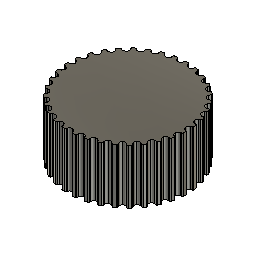
gear_35z (Autodesk Fusion 360 design; units mm, degrees)
Autodesk Fusion 360 part; units mm, degrees
sketch "Sketch1" plane through (0, 0, 0) normal (0, 0, 1) x (1, 0, 0) in component "gt2 pulley"
  circle A0 centre (0, 0) radius 11.1408 construction
  circle A1 centre (0, 0) radius 10.1368 construction
  line L0 (0, 0) -> (0, 11.1408) construction
  line L1 (0, 0) -> (0.9987, 11.096) construction
  line L2 (0, 0) -> (1.4093, 11.0514) construction
  circle A2 centre (0, 0) radius 10.8868 construction
  arc A3 (0.3788, 10.7429) -> (0.4362, 10.461) centre (1.3772, 10.7994) ccw
  circle A4 centre (0, 0) radius 10.7368 construction
  arc A5 (0.2321, 10.8844) -> (0, 10.8868) centre (0, 0) ccw
  arc A6 (0.3788, 10.7429) -> (0.2321, 10.8844) centre (0.229, 10.7344) ccw
  arc A7 (0.4362, 10.461) -> (0.9087, 10.096) centre (0.9584, 10.6488) ccw
  arc A8 (0, 10.8868) -> (-0.2321, 10.8844) centre (0, 0) ccw
  arc A9 (-0.2321, 10.8844) -> (-0.3788, 10.7429) centre (-0.229, 10.7344) ccw
  arc A10 (-0.4362, 10.461) -> (-0.3788, 10.7429) centre (-1.3772, 10.7994) ccw
  arc A11 (-0.9096, 10.096) -> (-0.4362, 10.461) centre (-0.9584, 10.6488) ccw
  arc A12 (0.9087, 10.096) -> (-0.9087, 10.096) centre (0, 0) ccw
  point P0 (1.3772, 10.7994)
  point P1 (0, 10.8868)
  dimension "d18" = 22.2817
  dimension "d19" = 5.143
  dimension "d22" = 1.004
  dimension "d24" = 0.75
  dimension "d26" = 1
  dimension "d27" = 0.15
  dimension "d28" = 0.15
  dimension "d47" = 0.555
  dimension "d52" = 3.812
  constraint coincident A0.centre A1.centre
  constraint coincident A0 L0.end
  constraint vertical L0
  constraint coincident A0 L1.end
  constraint coincident A0 L2.end
  constraint concentric A1 A2
  constraint coincident A1 A7.end
  constraint coincident L1 A7.end
  constraint coincident A2 P0
  constraint coincident L2 P0
  constraint coincident P0 A3.centre
  constraint coincident A2 P1
  constraint coincident L0 P1
  constraint concentric A2 A4
  constraint coincident P1 A5.end
  constraint coincident A4 A6.centre
  constraint coincident A3.start A6.start
  constraint tangent A3 A6
  constraint tangent A3 A7
  constraint symmetric L0 A7.end A12.end
  constraint symmetric L0 A3.start A9.end
  constraint symmetric L0 A3.end A10.start
  constraint symmetric L0 A3 A10
  constraint symmetric L0 A5.start A8.end
  constraint symmetric L0 P1 A5.end
  constraint symmetric L0 A5 A8
  constraint symmetric L0 A6 A9
  constraint symmetric L0 A7 A11
  constraint coincident A1 A11.start
  constraint tangent A1 A7
  constraint coincident L1 A7.centre
  measures "d18" diameter of A0
  measures "d19" angle of L0 L1
  measures "d22" distance of A0 A1
  measures "d24" distance of A1 A2
  measures "d26" radius of A3
  measures "d27" distance of A2 A4
  measures "d28" radius of A6
  measures "d47" radius of A7
extrude "Extrude1" add sketch "Sketch1" along normal blind 10 makes body 1
pattern_circular "C-Pattern1" count 35 over 360 about axis through (0, 0, 1.75) along (0, 0, 1) of bodies 1 makes body 2 at (-2.5021, 9.8232, 6.6667) makes body 3 at (-3.6568, 9.4543, 6.6667) makes body 4 at (-5.2861, 8.6494, 6.6667) makes body 5 at (-7.1863, 7.1494, 6.6667) makes body 6 at (-8.3473, 5.7513, 6.6667) makes body 7 at (-8.5697, 5.4144, 3.3333) makes body 8 at (-9.3988, 3.7972, 3.3333) makes body 9 at (-10.1156, 0.6559, 6.6667) makes body 10 at (-10.1216, -0.5563, 6.6667) makes body 11 at (-10.016, -1.5609, 3.3333) makes body 12 at (-9.0201, -4.6253, 6.6667) makes body 13 at (-8.4035, -5.6689, 6.6667) makes body 14 at (-6.8197, -7.4998, 6.6667) makes body 15 at (-5.371, -8.597, 6.6667) makes body 16 at (-5.0245, -8.804, 3.3333) makes body 17 at (-3.3717, -9.5597, 3.3333) makes body 18 at (-0.8074, -10.1046, 6.6667) makes body 19 at (1.0098, -10.0864, 6.6667) makes body 20 at (2.0087, -9.9358, 3.3333) makes body 21 at (5.0253, -8.8035, 6.6667) makes body 22 at (5.3718, -8.5965, 3.3333) makes body 23 at (6.8204, -7.4992, 3.3333) makes body 24 at (8.0498, -6.1608, 3.3333) makes body 25 at (9.5766, -3.3233, 6.6667) makes body 26 at (10.0161, -1.56, 6.6667) makes body 27 at (10.1307, -0.3533, 6.6667) makes body 28 at (9.9256, 2.0589, 6.6667) makes body 29 at (9.6088, 3.2289, 6.6667) makes body 30 at (8.5692, 5.4152, 6.6667) makes body 31 at (7.8616, 6.3993, 6.6667) makes body 32 at (6.12, 8.0809, 6.6667) makes body 33 at (5.7935, 8.3181, 3.3333) makes body 34 at (4.2151, 9.2189, 3.3333) makes body 35 at (1.7099, 9.9916, 6.6667)
sketch "Sketch2" plane through (0, 0, 10) normal (0, 0, 1) x (-1, 0, 0)
  arc A0 (-10.7151, 0.8603) -> (-10.863, 0.7202) centre (-10.7133, 0.7104) ccw
  arc A1 (-10.863, 0.7202) -> (-10.8838, 0.2564) centre (0, 0) ccw
  arc A2 (-10.8838, 0.2564) -> (-10.7491, 0.1036) centre (-10.7339, 0.2528) ccw
  arc A3 (-10.47, 0.0336) -> (-10.7491, 0.1036) centre (-10.8503, -0.8913) ccw
  arc A4 (-10.1266, -0.4548) -> (-10.47, 0.0336) centre (-10.6811, -0.4797) ccw
  arc A5 (-10.0451, 1.3607) -> (-10.1266, -0.4548) centre (0, 0) ccw
  arc A6 (-10.4309, 0.905) -> (-10.0451, 1.3607) centre (-10.5951, 1.4352) ccw
  arc A7 (-10.7151, 0.8603) -> (-10.4309, 0.905) centre (-10.7267, 1.8603) ccw
  circle A8 centre (0, 0) radius 10.1368
  constraint concentric A1 A8
extrude "Extrude2" add sketch "Sketch2" against normal blind 10 contours A5 A8 bodies 1 2 3 4 5 6 7 8 9 10 11 12 13 14 15 16 17 18 19 20 21 22 23 24 25 26 27 28 29 30 31 32 33 34 35
extrude "Extrude4" [suppressed] in component "gt2 pulley"
pattern_circular "C-Pattern7" [suppressed] in component "gt2 pulley"
extrude "Extrude3" [suppressed] in component "gt2 pulley"
pattern_circular "C-Pattern6" [suppressed] in component "gt2 pulley"
extrude "Extrude2'" [suppressed] in component "gt2 pulley"
pattern_circular "C-Pattern5" [suppressed] in component "gt2 pulley"
extrude "Extrude1'" [suppressed] in component "gt2 pulley"
pattern_circular "C-Pattern4" [suppressed] in component "gt2 pulley"
pattern_circular "C-Pattern3" [suppressed] in component "gt2 pulley"
pattern_circular "C-Pattern2" [suppressed] in component "gt2 pulley"
pattern_circular "C-Pattern1'" [suppressed] in component "gt2 pulley"
copy_body "Body->Comp1" [suppressed] in component "Component"
copy_body "Body->Comp2" [suppressed] in component "Component'"
copy_body "Body->Comp3" [suppressed] in component "Component''"
copy_body "Body->Comp4" [suppressed] in component "Component'''"
copy_body "Body->Comp5" [suppressed] in component "Component''''"
copy_body "Body->Comp6" [suppressed] in component "Component'''''"
copy_body "Body->Comp7" [suppressed] in component "Component''''''"
copy_body "Body->Comp8" [suppressed] in component "Component'''''''"
copy_body "Body->Comp9" [suppressed] in component "Component''''''''"
copy_body "Body->Comp10" [suppressed] in component "Component'''''''''"
copy_body "Body->Comp11" [suppressed] in component "Component''''''''''"
copy_body "Body->Comp12" [suppressed] in component "Component'''''''''''"
copy_body "Body->Comp13" [suppressed] in component "Component''''''''''''"
copy_body "Body->Comp14" [suppressed] in component "Component'''''''''''''"
copy_body "Body->Comp15" [suppressed] in component "Component''''''''''''''"
copy_body "Body->Comp16" [suppressed] in component "Component'''''''''''''''"
copy_body "Body->Comp17" [suppressed] in component "Component''''''''''''''''"
copy_body "Body->Comp18" [suppressed] in component "Component'''''''''''''''''"
copy_body "Body->Comp19" [suppressed] in component "Component''''''''''''''''''"
copy_body "Body->Comp20" [suppressed] in component "Component'''''''''''''''''''"
component "gt2 pulley" placed x (1, 0, 0) y (0, 1, 0) z (0, 0, 1) at (0, 0, 0)
equation "NumTeeth = 35" comment "min 20"
equation "ToothPitch = 2 mm"
equation "PullyDia = NumTeeth * ToothPitch / PI"
equation "ToothAng = ( ( 360 / NumTeeth ) * 1 deg )"
equation "TransOffsetAngle = ToothAng * 0.2"
equation "Sholulder_Radius = 0.15 mm"
equation "Root_Radius = 0.555 mm"
equation "TransRadius = 1 mm"
equation "ToolHeight = 0.75 mm"
equation "PLD = 0.254 mm"
equation "d18 = PullyDia"
equation "d19 = ToothAng / 2"
equation "d22 = PLD + ToolHeight"
equation "d24 = ToolHeight"
equation "d26 = TransRadius"
equation "d27 = Sholulder_Radius"
equation "d31 = NumTeeth"
equation "d33 = NumTeeth"
equation "d35 = NumTeeth"
equation "d37 = NumTeeth"
equation "d41 = NumTeeth"
equation "d45 = NumTeeth"
equation "d47 = Root_Radius"
equation "d50 = NumTeeth"
